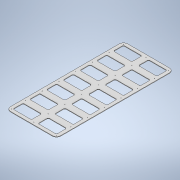
# Autodesk Inventor part: front_Box
Saved by Autodesk Inventor 2020 (Build 240168000, 168)
## iProperties
Created: 2020-07-08
Part Number: front_Box
Material: Generic
Document SubType Name: Modeling
Designer: gerac
Density: 1 g/cm^3
Appearance: Default
Author: gerac
Autodesk Inventor part; units mm, degrees
ref_plane "YZ Plane" through (0, 0, 0) normal (1, 0, 0) x (0, 1, 0)
ref_plane "XZ Plane" through (0, 0, 0) normal (0, 1, 0) x (-1, 0, 0)
ref_plane "XY Plane" through (0, 0, 0) normal (0, 0, 1) x (1, 0, 0)
sketch "Sketch1" plane through (0, 0, 0) normal (0, 1, 0) x (-1, 0, 0)
  line L0 (144, 336) -> (-144, 336)
  line L1 (-144, 336) -> (-144, -336)
  line L2 (-144, -336) -> (144, -336)
  line L3 (144, -336) -> (144, 336)
  line L4 (144, 336) -> (-144, -336) construction
  line L5 (-144, 336) -> (144, -336) construction
  line L6 (-24, 317) -> (-19, 312)
  line L7 (-19, 264) -> (-24, 259)
  line L8 (-125, 264) -> (-120, 259)
  line L9 (-120, 317) -> (-125, 312)
  line L10 (-19, 312) -> (-19, 264)
  line L11 (-24, 259) -> (-120, 259)
  line L12 (-24, 317) -> (-120, 317)
  line L13 (-125, 312) -> (-125, 264)
  line L14 (-24, 221) -> (-120, 221)
  line L15 (-24, 221) -> (-19, 216)
  line L16 (-19, 216) -> (-19, 168)
  line L17 (-24, 163) -> (-120, 163)
  line L18 (-19, 168) -> (-24, 163)
  line L19 (-125, 168) -> (-120, 163)
  line L20 (-125, 216) -> (-125, 168)
  line L21 (-120, 221) -> (-125, 216)
  line L22 (-24, 125) -> (-120, 125)
  line L23 (-24, 125) -> (-19, 120)
  line L24 (-19, 120) -> (-19, 72)
  line L25 (-24, 67) -> (-120, 67)
  line L26 (-19, 72) -> (-24, 67)
  line L27 (-125, 72) -> (-120, 67)
  line L28 (-125, 120) -> (-125, 72)
  line L29 (-120, 125) -> (-125, 120)
  line L30 (-24, 29) -> (-120, 29)
  line L31 (-24, 29) -> (-19, 24)
  line L32 (-19, 24) -> (-19, -24)
  line L33 (-24, -29) -> (-120, -29)
  line L34 (-19, -24) -> (-24, -29)
  line L35 (-125, -24) -> (-120, -29)
  line L36 (-125, 24) -> (-125, -24)
  line L37 (-120, 29) -> (-125, 24)
  line L38 (-24, -67) -> (-120, -67)
  line L39 (-24, -67) -> (-19, -72)
  line L40 (-19, -72) -> (-19, -120)
  line L41 (-24, -125) -> (-120, -125)
  line L42 (-19, -120) -> (-24, -125)
  line L43 (-125, -120) -> (-120, -125)
  line L44 (-125, -72) -> (-125, -120)
  line L45 (-120, -67) -> (-125, -72)
  line L46 (-24, -163) -> (-120, -163)
  line L47 (-24, -163) -> (-19, -168)
  line L48 (-19, -168) -> (-19, -216)
  line L49 (-24, -221) -> (-120, -221)
  line L50 (-19, -216) -> (-24, -221)
  line L51 (-125, -216) -> (-120, -221)
  line L52 (-125, -168) -> (-125, -216)
  line L53 (-120, -163) -> (-125, -168)
  line L54 (-24, -259) -> (-120, -259)
  line L55 (-24, -259) -> (-19, -264)
  line L56 (-19, -264) -> (-19, -312)
  line L57 (-24, -317) -> (-120, -317)
  line L58 (-19, -312) -> (-24, -317)
  line L59 (-125, -312) -> (-120, -317)
  line L60 (-125, -264) -> (-125, -312)
  line L61 (-120, -259) -> (-125, -264)
  line L62 (120, 317) -> (24, 317)
  line L63 (120, 317) -> (125, 312)
  line L64 (125, 312) -> (125, 264)
  line L65 (120, 259) -> (24, 259)
  line L66 (125, 264) -> (120, 259)
  line L67 (19, 264) -> (24, 259)
  line L68 (19, 312) -> (19, 264)
  line L69 (24, 317) -> (19, 312)
  line L70 (120, 221) -> (24, 221)
  line L71 (120, 221) -> (125, 216)
  line L72 (125, 216) -> (125, 168)
  line L73 (120, 163) -> (24, 163)
  line L74 (125, 168) -> (120, 163)
  line L75 (19, 168) -> (24, 163)
  line L76 (19, 216) -> (19, 168)
  line L77 (24, 221) -> (19, 216)
  line L78 (120, 125) -> (24, 125)
  line L79 (120, 125) -> (125, 120)
  line L80 (125, 120) -> (125, 72)
  line L81 (120, 67) -> (24, 67)
  line L82 (125, 72) -> (120, 67)
  line L83 (19, 72) -> (24, 67)
  line L84 (19, 120) -> (19, 72)
  line L85 (24, 125) -> (19, 120)
  line L86 (120, 29) -> (24, 29)
  line L87 (120, 29) -> (125, 24)
  line L88 (125, 24) -> (125, -24)
  line L89 (120, -29) -> (24, -29)
  line L90 (125, -24) -> (120, -29)
  line L91 (19, -24) -> (24, -29)
  line L92 (19, 24) -> (19, -24)
  line L93 (24, 29) -> (19, 24)
  line L94 (120, -67) -> (24, -67)
  line L95 (120, -67) -> (125, -72)
  line L96 (125, -72) -> (125, -120)
  line L97 (120, -125) -> (24, -125)
  line L98 (125, -120) -> (120, -125)
  line L99 (19, -120) -> (24, -125)
  line L100 (19, -72) -> (19, -120)
  line L101 (24, -67) -> (19, -72)
  line L102 (120, -163) -> (24, -163)
  line L103 (120, -163) -> (125, -168)
  line L104 (125, -168) -> (125, -216)
  line L105 (120, -221) -> (24, -221)
  line L106 (125, -216) -> (120, -221)
  line L107 (19, -216) -> (24, -221)
  line L108 (19, -168) -> (19, -216)
  line L109 (24, -163) -> (19, -168)
  line L110 (120, -259) -> (24, -259)
  line L111 (120, -259) -> (125, -264)
  line L112 (125, -264) -> (125, -312)
  line L113 (120, -317) -> (24, -317)
  line L114 (125, -312) -> (120, -317)
  line L115 (19, -312) -> (24, -317)
  line L116 (19, -264) -> (19, -312)
  line L117 (24, -259) -> (19, -264)
  line L118 (-125.2, 263.9172) -> (-125.2, 312.0828)
  line L119 (-125.2, 312.0828) -> (-120.0828, 317.2)
  line L120 (-120.0828, 317.2) -> (-23.9172, 317.2)
  line L121 (-23.9172, 317.2) -> (-18.8, 312.0828)
  line L122 (-18.8, 312.0828) -> (-18.8, 263.9172)
  line L123 (-18.8, 263.9172) -> (-23.9172, 258.8)
  line L124 (-23.9172, 258.8) -> (-120.0828, 258.8)
  line L125 (-120.0828, 258.8) -> (-125.2, 263.9172)
  line L126 (125.2, 312.0828) -> (125.2, 263.9172)
  line L127 (125.2, 263.9172) -> (120.0828, 258.8)
  line L128 (120.0828, 258.8) -> (23.9172, 258.8)
  line L129 (23.9172, 258.8) -> (18.8, 263.9172)
  line L130 (18.8, 263.9172) -> (18.8, 312.0828)
  line L131 (18.8, 312.0828) -> (23.9172, 317.2)
  line L132 (23.9172, 317.2) -> (120.0828, 317.2)
  line L133 (120.0828, 317.2) -> (125.2, 312.0828)
  line L134 (-18.8, 216.0828) -> (-18.8, 167.9172)
  line L135 (-18.8, 167.9172) -> (-23.9172, 162.8)
  line L136 (-23.9172, 162.8) -> (-120.0828, 162.8)
  line L137 (-120.0828, 162.8) -> (-125.2, 167.9172)
  line L138 (-125.2, 167.9172) -> (-125.2, 216.0828)
  line L139 (-125.2, 216.0828) -> (-120.0828, 221.2)
  line L140 (-120.0828, 221.2) -> (-23.9172, 221.2)
  line L141 (-23.9172, 221.2) -> (-18.8, 216.0828)
  line L142 (125.2, 216.0828) -> (125.2, 167.9172)
  line L143 (125.2, 167.9172) -> (120.0828, 162.8)
  line L144 (120.0828, 162.8) -> (23.9172, 162.8)
  line L145 (23.9172, 162.8) -> (18.8, 167.9172)
  line L146 (18.8, 167.9172) -> (18.8, 216.0828)
  line L147 (18.8, 216.0828) -> (23.9172, 221.2)
  line L148 (23.9172, 221.2) -> (120.0828, 221.2)
  line L149 (120.0828, 221.2) -> (125.2, 216.0828)
  line L150 (-18.8, 120.0828) -> (-18.8, 71.9172)
  line L151 (-18.8, 71.9172) -> (-23.9172, 66.8)
  line L152 (-23.9172, 66.8) -> (-120.0828, 66.8)
  line L153 (-120.0828, 66.8) -> (-125.2, 71.9172)
  line L154 (-125.2, 71.9172) -> (-125.2, 120.0828)
  line L155 (-125.2, 120.0828) -> (-120.0828, 125.2)
  line L156 (-120.0828, 125.2) -> (-23.9172, 125.2)
  line L157 (-23.9172, 125.2) -> (-18.8, 120.0828)
  line L158 (125.2, 120.0828) -> (125.2, 71.9172)
  line L159 (125.2, 71.9172) -> (120.0828, 66.8)
  line L160 (120.0828, 66.8) -> (23.9172, 66.8)
  line L161 (23.9172, 66.8) -> (18.8, 71.9172)
  line L162 (18.8, 71.9172) -> (18.8, 120.0828)
  line L163 (18.8, 120.0828) -> (23.9172, 125.2)
  line L164 (23.9172, 125.2) -> (120.0828, 125.2)
  line L165 (120.0828, 125.2) -> (125.2, 120.0828)
  line L166 (-18.8, 24.0828) -> (-18.8, -24.0828)
  line L167 (-18.8, -24.0828) -> (-23.9172, -29.2)
  line L168 (-23.9172, -29.2) -> (-120.0828, -29.2)
  line L169 (-120.0828, -29.2) -> (-125.2, -24.0828)
  line L170 (-125.2, -24.0828) -> (-125.2, 24.0828)
  line L171 (-125.2, 24.0828) -> (-120.0828, 29.2)
  line L172 (-120.0828, 29.2) -> (-23.9172, 29.2)
  line L173 (-23.9172, 29.2) -> (-18.8, 24.0828)
  line L174 (125.2, 24.0828) -> (125.2, -24.0828)
  line L175 (125.2, -24.0828) -> (120.0828, -29.2)
  line L176 (120.0828, -29.2) -> (23.9172, -29.2)
  line L177 (23.9172, -29.2) -> (18.8, -24.0828)
  line L178 (18.8, -24.0828) -> (18.8, 24.0828)
  line L179 (18.8, 24.0828) -> (23.9172, 29.2)
  line L180 (23.9172, 29.2) -> (120.0828, 29.2)
  line L181 (120.0828, 29.2) -> (125.2, 24.0828)
  line L182 (-18.8, -71.9172) -> (-18.8, -120.0828)
  line L183 (-18.8, -120.0828) -> (-23.9172, -125.2)
  line L184 (-23.9172, -125.2) -> (-120.0828, -125.2)
  line L185 (-120.0828, -125.2) -> (-125.2, -120.0828)
  line L186 (-125.2, -120.0828) -> (-125.2, -71.9172)
  line L187 (-125.2, -71.9172) -> (-120.0828, -66.8)
  line L188 (-120.0828, -66.8) -> (-23.9172, -66.8)
  line L189 (-23.9172, -66.8) -> (-18.8, -71.9172)
  line L190 (125.2, -71.9172) -> (125.2, -120.0828)
  line L191 (125.2, -120.0828) -> (120.0828, -125.2)
  line L192 (120.0828, -125.2) -> (23.9172, -125.2)
  line L193 (23.9172, -125.2) -> (18.8, -120.0828)
  line L194 (18.8, -120.0828) -> (18.8, -71.9172)
  line L195 (18.8, -71.9172) -> (23.9172, -66.8)
  line L196 (23.9172, -66.8) -> (120.0828, -66.8)
  line L197 (120.0828, -66.8) -> (125.2, -71.9172)
  line L198 (-18.8, -167.9172) -> (-18.8, -216.0828)
  line L199 (-18.8, -216.0828) -> (-23.9172, -221.2)
  line L200 (-23.9172, -221.2) -> (-120.0828, -221.2)
  line L201 (-120.0828, -221.2) -> (-125.2, -216.0828)
  line L202 (-125.2, -216.0828) -> (-125.2, -167.9172)
  line L203 (-125.2, -167.9172) -> (-120.0828, -162.8)
  line L204 (-120.0828, -162.8) -> (-23.9172, -162.8)
  line L205 (-23.9172, -162.8) -> (-18.8, -167.9172)
  line L206 (125.2, -167.9172) -> (125.2, -216.0828)
  line L207 (125.2, -216.0828) -> (120.0828, -221.2)
  line L208 (120.0828, -221.2) -> (23.9172, -221.2)
  line L209 (23.9172, -221.2) -> (18.8, -216.0828)
  line L210 (18.8, -216.0828) -> (18.8, -167.9172)
  line L211 (18.8, -167.9172) -> (23.9172, -162.8)
  line L212 (23.9172, -162.8) -> (120.0828, -162.8)
  line L213 (120.0828, -162.8) -> (125.2, -167.9172)
  line L214 (-18.8, -263.9172) -> (-18.8, -312.0828)
  line L215 (-18.8, -312.0828) -> (-23.9172, -317.2)
  line L216 (-23.9172, -317.2) -> (-120.0828, -317.2)
  line L217 (-120.0828, -317.2) -> (-125.2, -312.0828)
  line L218 (-125.2, -312.0828) -> (-125.2, -263.9172)
  line L219 (-125.2, -263.9172) -> (-120.0828, -258.8)
  line L220 (-120.0828, -258.8) -> (-23.9172, -258.8)
  line L221 (-23.9172, -258.8) -> (-18.8, -263.9172)
  line L222 (125.2, -263.9172) -> (125.2, -312.0828)
  line L223 (125.2, -312.0828) -> (120.0828, -317.2)
  line L224 (120.0828, -317.2) -> (23.9172, -317.2)
  line L225 (23.9172, -317.2) -> (18.8, -312.0828)
  line L226 (18.8, -312.0828) -> (18.8, -263.9172)
  line L227 (18.8, -263.9172) -> (23.9172, -258.8)
  line L228 (23.9172, -258.8) -> (120.0828, -258.8)
  line L229 (120.0828, -258.8) -> (125.2, -263.9172)
  point P0 (0, 0)
  dimension "d0" = 288
  dimension "d1" = 672
  dimension "d19" = 19
  dimension "d30" = 48
  dimension "d31" = 58
  dimension "d32" = 96
  dimension "d33" = 106
  dimension "d34" = 19
  dimension "d38" = 5
  dimension "d39" = 5
  dimension "d40" = 5
  dimension "d41" = 5
  dimension "d42" = 5
  dimension "d43" = 5
  dimension "d44" = 5
  dimension "d47" = 96
  dimension "d50" = 144
  dimension "d161" = 0.2
  dimension "d162" = 0.2
  dimension "d163" = 0.2
  dimension "d164" = 0.2
  dimension "d165" = 0.2
  dimension "d166" = 0.2
  dimension "d167" = 0.2
  dimension "d168" = 0.2
  dimension "d171" = 144
  dimension "d174" = 96
  constraints: 460 end point, 14 point on line, 9 parallel, 4 vertical, 3 horizontal, 2 midpoint, 2 perpendicular, 429 other
  measures "d0" distance of L2.end L1.end
  measures "d1" distance of L1.end L0.end
  measures "d19" distance between parallel lines of L0 L12
  measures "d30" distance of L6.end L10.end
  measures "d31" distance between parallel lines of L11 L12
  measures "d32" distance of L7.end L8.end
  measures "d33" distance between parallel lines of L13 L10
  measures "d34" distance between parallel lines of L1 L13
  measures "d38" horizontal distance of L8.start L8.end
  measures "d39" horizontal distance of L8.start L8.end
  measures "d40" horizontal distance of L9.start L9.end
  measures "d41" horizontal distance of L9.start L9.end
  measures "d42" horizontal distance of L6.start L6.end
  measures "d43" horizontal distance of L6.start L6.end
  measures "d44" horizontal distance of L7.start L7.end
  measures "d47" distance of L6.start L14.start
  measures "d50" distance of L6.start L62.start
  measures "d161" distance between parallel lines of L122 L10
  measures "d162" distance between parallel lines of L7 L123
  measures "d163" distance between parallel lines of L11 L124
  measures "d164" distance between parallel lines of L8 L125
  measures "d165" distance between parallel lines of L13 L118
  measures "d166" distance between parallel lines of L9 L119
  measures "d167" distance between parallel lines of L12 L120
  measures "d168" distance between parallel lines of L121 L6
  measures "d171" distance of L121.end L126.start
  measures "d174" distance of L121.end L134.start
extrude "Extrusion2" add sketch "Sketch1" along normal blind 3 contours L3 L2 L1 L0 | L118 L119 L120 L121 L122 L123 L124 L125 | L126 L127 L128 L129 L130 L131 L132 L133 | L134 L135 L136 L137 L138 L139 L140 L141 | L142 L143 L144 L145 L146 L147 L148 L149 | L150 L151 L152 L153 L154 L155 L156 L157 | L158 L159 L160 L161 L162 L163 L164 L165 | L166 L167 L168 L169 L170 L171 L172 L173 | L174 L175 L176 L177 L178 L179 L180 L181 | L182 L183 L184 L185 L186 L187 L188 L189 | L190 L191 L192 L193 L194 L195 L196 L197 | L198 L199 L200 L201 L202 L203 L204 L205 | L206 L207 L208 L209 L210 L211 L212 L213 | L214 L215 L216 L217 L218 L219 L220 L221 | L222 L223 L224 L225 L226 L227 L228 L229
fillet "Fillet1" radius 24 4 edges at (-144, 1.5, 336) (-144, 1.5, -336) (144, 1.5, 336) (144, 1.5, -336)
sketch "Sketch5" plane through (0, 3, 0) normal (0, 1, 0) x (1, 0, 0)
  circle A0 centre (130, -322) radius 1.25
  line L0 (144, -312) -> (144, 312) projected
  line L1 (-120, -336) -> (120, -336) projected
  circle A1 centre (0, -322) radius 1.25
  circle A2 centre (-130, -322) radius 1.25
  circle A3 centre (130, 322) radius 1.25
  circle A4 centre (0, 322) radius 1.25
  circle A5 centre (-130, 322) radius 1.25
  circle A6 centre (130, -240) radius 1.25
  line L2 (24, -259) -> (120, -259) projected
  circle A7 centre (0, -240) radius 1.25
  circle A8 centre (-130, -240) radius 1.25
  circle A9 centre (130, -144) radius 1.25
  circle A10 centre (0, -144) radius 1.25
  circle A11 centre (-130, -144) radius 1.25
  circle A12 centre (130, -48) radius 1.25
  circle A13 centre (0, -48) radius 1.25
  circle A14 centre (-130, -48) radius 1.25
  circle A15 centre (130, 48) radius 1.25
  circle A16 centre (0, 48) radius 1.25
  circle A17 centre (-130, 48) radius 1.25
  circle A18 centre (130, 144) radius 1.25
  circle A19 centre (0, 144) radius 1.25
  circle A20 centre (-130, 144) radius 1.25
  circle A21 centre (130, 240) radius 1.25
  circle A22 centre (0, 240) radius 1.25
  circle A23 centre (-130, 240) radius 1.25
  point P0 (0, 0)
  dimension "d137" = 2.5
  dimension "d138" = 14
  dimension "d139" = 14
  dimension "d142" = 130
  dimension "d145" = 644
  dimension "d148" = 2.5
  dimension "d149" = 14
  dimension "d150" = 19
  dimension "d153" = 130
  dimension "d156" = 96
  constraints: 24 centre point, 2 horizontal, 2 vertical, 44 other
  measures "d137" diameter of A0
  measures "d138" distance from line of L0 A0.centre
  measures "d139" distance from line of L1 A0.centre
  measures "d142" distance of A0.centre A1.centre
  measures "d145" distance of A0.centre A3.centre
  measures "d148" diameter of A6
  measures "d149" distance from line of L0 A6.centre
  measures "d150" distance from line of L2 A6.centre
  measures "d153" distance of A6.centre A7.centre
  measures "d156" distance of A6.centre A9.centre
extrude "Extrusion6" cut sketch "Sketch5" against normal blind 3
sketch "Sketch7" plane through (0, 3, 0) normal (0, 1, 0) x (1, 0, 0)
  line L0 (23.9172, -317.2) -> (18.8, -312.0828)
  line L1 (18.8, -312.0828) -> (18.8, -263.9172)
  line L2 (18.8, -263.9172) -> (23.9172, -258.8)
  line L3 (23.9172, -258.8) -> (120.0828, -258.8)
  line L4 (120.0828, -258.8) -> (125.2, -263.9172)
  line L5 (125.2, -263.9172) -> (125.2, -312.0828)
  line L6 (125.2, -312.0828) -> (120.0828, -317.2)
  line L7 (120.0828, -317.2) -> (23.9172, -317.2)
  line L8 (19, -312) -> (19, -264) projected
  line L9 (19, -264) -> (24, -259) projected
  line L10 (24, -259) -> (120, -259) projected
  line L11 (24, -317) -> (19, -312) projected
  line L12 (120, -317) -> (24, -317) projected
  line L13 (125, -264) -> (125, -312) projected
  line L14 (125, -312) -> (120, -317) projected
  line L15 (120, -259) -> (125, -264) projected
  line L16 (-125.2, -312.0828) -> (-125.2, -263.9172)
  line L17 (-125.2, -263.9172) -> (-120.0828, -258.8)
  line L18 (-120.0828, -258.8) -> (-23.9172, -258.8)
  line L19 (-23.9172, -258.8) -> (-18.8, -263.9172)
  line L20 (-18.8, -263.9172) -> (-18.8, -312.0828)
  line L21 (-23.9172, -317.2) -> (-120.0828, -317.2)
  line L22 (-18.8, -312.0828) -> (-23.9172, -317.2)
  line L23 (-120.0828, -317.2) -> (-125.2, -312.0828)
  line L24 (18.8, -216.0828) -> (18.8, -167.9172)
  line L25 (18.8, -167.9172) -> (23.9172, -162.8)
  line L26 (23.9172, -162.8) -> (120.0828, -162.8)
  line L27 (120.0828, -162.8) -> (125.2, -167.9172)
  line L28 (125.2, -167.9172) -> (125.2, -216.0828)
  line L29 (120.0828, -221.2) -> (23.9172, -221.2)
  line L30 (125.2, -216.0828) -> (120.0828, -221.2)
  line L31 (23.9172, -221.2) -> (18.8, -216.0828)
  line L32 (-125.2, -216.0828) -> (-125.2, -167.9172)
  line L33 (-125.2, -167.9172) -> (-120.0828, -162.8)
  line L34 (-120.0828, -162.8) -> (-23.9172, -162.8)
  line L35 (-23.9172, -162.8) -> (-18.8, -167.9172)
  line L36 (-18.8, -167.9172) -> (-18.8, -216.0828)
  line L37 (-23.9172, -221.2) -> (-120.0828, -221.2)
  line L38 (-18.8, -216.0828) -> (-23.9172, -221.2)
  line L39 (-120.0828, -221.2) -> (-125.2, -216.0828)
  line L40 (18.8, -120.0828) -> (18.8, -71.9172)
  line L41 (18.8, -71.9172) -> (23.9172, -66.8)
  line L42 (23.9172, -66.8) -> (120.0828, -66.8)
  line L43 (120.0828, -66.8) -> (125.2, -71.9172)
  line L44 (125.2, -71.9172) -> (125.2, -120.0828)
  line L45 (120.0828, -125.2) -> (23.9172, -125.2)
  line L46 (125.2, -120.0828) -> (120.0828, -125.2)
  line L47 (23.9172, -125.2) -> (18.8, -120.0828)
  line L48 (-125.2, -120.0828) -> (-125.2, -71.9172)
  line L49 (-125.2, -71.9172) -> (-120.0828, -66.8)
  line L50 (-120.0828, -66.8) -> (-23.9172, -66.8)
  line L51 (-23.9172, -66.8) -> (-18.8, -71.9172)
  line L52 (-18.8, -71.9172) -> (-18.8, -120.0828)
  line L53 (-23.9172, -125.2) -> (-120.0828, -125.2)
  line L54 (-18.8, -120.0828) -> (-23.9172, -125.2)
  line L55 (-120.0828, -125.2) -> (-125.2, -120.0828)
  line L56 (18.8, -24.0828) -> (18.8, 24.0828)
  line L57 (18.8, 24.0828) -> (23.9172, 29.2)
  line L58 (23.9172, 29.2) -> (120.0828, 29.2)
  line L59 (120.0828, 29.2) -> (125.2, 24.0828)
  line L60 (125.2, 24.0828) -> (125.2, -24.0828)
  line L61 (120.0828, -29.2) -> (23.9172, -29.2)
  line L62 (125.2, -24.0828) -> (120.0828, -29.2)
  line L63 (23.9172, -29.2) -> (18.8, -24.0828)
  line L64 (-125.2, -24.0828) -> (-125.2, 24.0828)
  line L65 (-125.2, 24.0828) -> (-120.0828, 29.2)
  line L66 (-120.0828, 29.2) -> (-23.9172, 29.2)
  line L67 (-23.9172, 29.2) -> (-18.8, 24.0828)
  line L68 (-18.8, 24.0828) -> (-18.8, -24.0828)
  line L69 (-23.9172, -29.2) -> (-120.0828, -29.2)
  line L70 (-18.8, -24.0828) -> (-23.9172, -29.2)
  line L71 (-120.0828, -29.2) -> (-125.2, -24.0828)
  line L72 (18.8, 71.9172) -> (18.8, 120.0828)
  line L73 (18.8, 120.0828) -> (23.9172, 125.2)
  line L74 (23.9172, 125.2) -> (120.0828, 125.2)
  line L75 (120.0828, 125.2) -> (125.2, 120.0828)
  line L76 (125.2, 120.0828) -> (125.2, 71.9172)
  line L77 (120.0828, 66.8) -> (23.9172, 66.8)
  line L78 (125.2, 71.9172) -> (120.0828, 66.8)
  line L79 (23.9172, 66.8) -> (18.8, 71.9172)
  line L80 (-125.2, 71.9172) -> (-125.2, 120.0828)
  line L81 (-125.2, 120.0828) -> (-120.0828, 125.2)
  line L82 (-120.0828, 125.2) -> (-23.9172, 125.2)
  line L83 (-23.9172, 125.2) -> (-18.8, 120.0828)
  line L84 (-18.8, 120.0828) -> (-18.8, 71.9172)
  line L85 (-23.9172, 66.8) -> (-120.0828, 66.8)
  line L86 (-18.8, 71.9172) -> (-23.9172, 66.8)
  line L87 (-120.0828, 66.8) -> (-125.2, 71.9172)
  line L88 (18.8, 167.9172) -> (18.8, 216.0828)
  line L89 (18.8, 216.0828) -> (23.9172, 221.2)
  line L90 (23.9172, 221.2) -> (120.0828, 221.2)
  line L91 (120.0828, 221.2) -> (125.2, 216.0828)
  line L92 (125.2, 216.0828) -> (125.2, 167.9172)
  line L93 (120.0828, 162.8) -> (23.9172, 162.8)
  line L94 (125.2, 167.9172) -> (120.0828, 162.8)
  line L95 (23.9172, 162.8) -> (18.8, 167.9172)
  line L96 (-125.2, 167.9172) -> (-125.2, 216.0828)
  line L97 (-125.2, 216.0828) -> (-120.0828, 221.2)
  line L98 (-120.0828, 221.2) -> (-23.9172, 221.2)
  line L99 (-23.9172, 221.2) -> (-18.8, 216.0828)
  line L100 (-18.8, 216.0828) -> (-18.8, 167.9172)
  line L101 (-23.9172, 162.8) -> (-120.0828, 162.8)
  line L102 (-18.8, 167.9172) -> (-23.9172, 162.8)
  line L103 (-120.0828, 162.8) -> (-125.2, 167.9172)
  line L104 (18.8, 263.9172) -> (18.8, 312.0828)
  line L105 (18.8, 312.0828) -> (23.9172, 317.2)
  line L106 (23.9172, 317.2) -> (120.0828, 317.2)
  line L107 (120.0828, 317.2) -> (125.2, 312.0828)
  line L108 (125.2, 312.0828) -> (125.2, 263.9172)
  line L109 (120.0828, 258.8) -> (23.9172, 258.8)
  line L110 (125.2, 263.9172) -> (120.0828, 258.8)
  line L111 (23.9172, 258.8) -> (18.8, 263.9172)
  line L112 (-125.2, 263.9172) -> (-125.2, 312.0828)
  line L113 (-125.2, 312.0828) -> (-120.0828, 317.2)
  line L114 (-120.0828, 317.2) -> (-23.9172, 317.2)
  line L115 (-23.9172, 317.2) -> (-18.8, 312.0828)
  line L116 (-18.8, 312.0828) -> (-18.8, 263.9172)
  line L117 (-23.9172, 258.8) -> (-120.0828, 258.8)
  line L118 (-18.8, 263.9172) -> (-23.9172, 258.8)
  line L119 (-120.0828, 258.8) -> (-125.2, 263.9172)
  point P0 (0, 0)
  dimension "d177" = 0.2
  dimension "d178" = 0.2
  dimension "d179" = 0.2
  dimension "d180" = 0.2
  dimension "d181" = 0.2
  dimension "d182" = 0.2
  dimension "d183" = 0.2
  dimension "d184" = 0.2
  dimension "d189" = 144
  dimension "d192" = 96
  constraints: 224 end point, 8 parallel, 2 horizontal, 2 perpendicular, 1 collinear, 1 vertical, 207 other
  measures "d177" distance between parallel lines of L8 L1
  measures "d178" distance between parallel lines of L9 L2
  measures "d179" distance between parallel lines of L10 L3
  measures "d180" distance between parallel lines of L11 L0
  measures "d181" distance between parallel lines of L12 L7
  measures "d182" distance between parallel lines of L14 L6
  measures "d183" distance between parallel lines of L13 L5
  measures "d184" distance between parallel lines of L15 L4
  measures "d189" distance of L0.end L16.start
  measures "d192" distance of L0.end L24.start
extrude "Extrusion8" cut sketch "Sketch7" against normal blind 3
equation "\"d162\" = d161"
equation "\"d163\" = d161"
equation "\"d164\" = d161"
equation "\"d165\" = d161"
equation "\"d166\" = d161"
equation "\"d167\" = d161"
equation "\"d168\" = d161"
equation "\"d178\" = d177"
equation "\"d179\" = d177"
equation "\"d180\" = d177"
equation "\"d181\" = d177"
equation "\"d182\" = d177"
equation "\"d183\" = d177"
equation "\"d184\" = d177"
body "Solid2"
